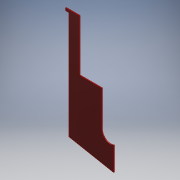
# Autodesk Inventor part: PolyCarb Cover
Saved by Autodesk Inventor 2019.4 (Build 234330000, 330)
## iProperties
Created: 2020-01-29
Part Number: PolyCarb Cover
Material: Polycarbonate, Smoke
Document SubType Name: Modeling
Designer: admin
Density: 1.2 g/cm^3
Appearance: Red
Author: admin
Autodesk Inventor part; units mm, degrees
ref_plane "YZ Plane" through (0, 0, 0) normal (1, 0, 0) x (0, 1, 0)
ref_plane "XZ Plane" through (0, 0, 0) normal (0, 1, 0) x (-1, 0, 0)
ref_plane "XY Plane" through (0, 0, 0) normal (0, 0, 1) x (1, 0, 0)
sketch "Sketch1" plane through (0, 0, 0) normal (0, 0, 1) x (1, 0, 0)
  line L0 (20, 110) -> (280, 60)
  line L1 (280, 60) -> (280, 197.1742)
  arc A0 (210, 243) -> (280, 197.1742) centre (260, 243) ccw
  line L2 (210, 243) -> (210, 450)
  line L3 (210, 450) -> (80, 450)
  line L4 (80, 450) -> (80, 750)
  line L5 (80, 750) -> (0, 750)
  line L6 (0, 750) -> (0, 0) projected
  line L7 (0, 750) -> (0, 735.9771)
  line L8 (0, 735.9771) -> (20, 735.9771)
  line L9 (20, 735.9771) -> (20, 110)
  dimension "d3" = 300
  dimension "d4" = 80
  dimension "d5" = 130
  dimension "d6" = 50
  dimension "d7" = 260
  dimension "d8" = 20
  dimension "d9" = 50
  dimension "d10" = 110
  dimension "d11" = 183
  constraints: 18 end point, 3 perpendicular, 3 vertical, 2 point on circle, 1 centre point, 1 horizontal, 1 point on line, 1 tangent
  measures "d3" distance of L3.end L4.end
  measures "d4" distance of L4.end L5.end
  measures "d5" distance of L2.end L3.end
  measures "d6" radius of A0
  measures "d7" distance between parallel lines of L9 L1
  measures "d8" distance of L7.end L8.end
  measures "d9" vertical distance of L0.start L0.end
  measures "d10" vertical distance of L0.start L6.end
  measures "d11" vertical distance of L0.end A0.centre
extrude "Extrusion1" add sketch "Sketch1" along normal blind 5
body "Solid1"
